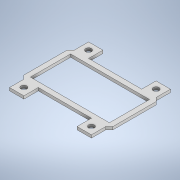
# Autodesk Inventor part: Spark MAX Holder Bottom
Saved by Autodesk Inventor 2020 (Build 240168000, 168)
## iProperties
Created: 2020-01-25
Part Number: Spark MAX Holder Bottom
Material: Generic
Document SubType Name: Modeling
Designer: 1twwarber
Density: 1 g/cm^3
Appearance: Default
Author: 1twwarber
Autodesk Inventor part; units mm, degrees
ref_plane "YZ Plane" through (0, 0, 0) normal (1, 0, 0) x (0, 1, 0)
ref_plane "XZ Plane" through (0, 0, 0) normal (0, 1, 0) x (-1, 0, 0)
ref_plane "XY Plane" through (0, 0, 0) normal (0, 0, 1) x (1, 0, 0)
sketch "Sketch1" plane through (0, 0, 0) normal (0, 1, 0) x (-1, 0, 0)
  line L0 (78.74, -3.175) -> (78.74, -41.275)
  line L1 (0, -41.275) -> (0, -3.175)
  line L2 (74.295, -4.445) -> (4.445, -4.445)
  line L3 (4.445, -4.445) -> (4.445, -40.005)
  line L4 (4.445, -40.005) -> (74.295, -40.005)
  line L5 (74.295, -40.005) -> (74.295, -4.445)
  line L6 (78.74, -3.175) -> (75.565, 0)
  line L7 (78.74, -41.275) -> (75.565, -44.45)
  line L8 (3.175, -44.45) -> (0, -41.275)
  line L9 (0, -3.175) -> (3.175, 0)
  line L10 (62.865, 0) -> (62.865, 12.7)
  line L11 (62.865, 12.7) -> (75.565, 12.7)
  line L12 (75.565, 12.7) -> (75.565, 0)
  line L13 (62.865, -44.45) -> (62.865, -57.15)
  line L14 (62.865, -57.15) -> (75.565, -57.15)
  line L15 (75.565, -57.15) -> (75.565, -44.45)
  line L16 (15.875, -44.45) -> (15.875, -57.15)
  line L17 (15.875, -57.15) -> (3.175, -57.15)
  line L18 (3.175, -57.15) -> (3.175, -44.45)
  line L19 (15.875, 0) -> (15.875, 12.7)
  line L20 (15.875, 12.7) -> (3.175, 12.7)
  line L21 (3.175, 12.7) -> (3.175, 0)
  line L22 (62.865, 0) -> (15.875, 0)
  line L23 (62.865, -44.45) -> (15.875, -44.45)
  circle A0 centre (69.215, 6.35) radius 2.54
  circle A1 centre (9.525, -50.8) radius 2.54
  circle A2 centre (9.525, 6.35) radius 2.54
  circle A3 centre (69.215, -50.8) radius 2.54
  constraints: 48 end point, 8 parallel, 4 centre point, 2 horizontal, 1 perpendicular
extrude "Extrusion1" add sketch "Sketch1" along normal blind 2.54
body "Solid1"
